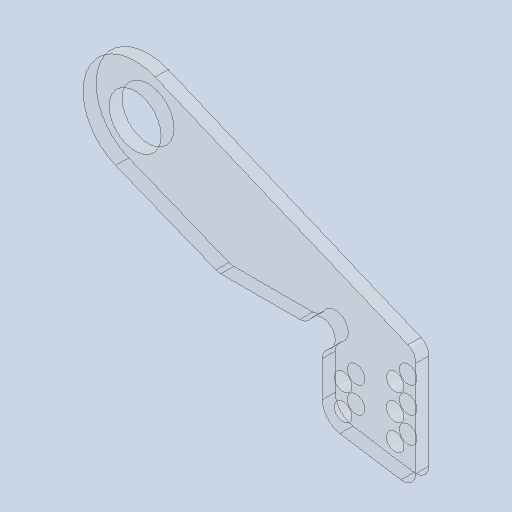
# Autodesk Inventor part: IntakePoly
Saved by Autodesk Inventor 2023 (Build 270158000, 158)
## iProperties
Created: 2022-11-06
Part Number: IntakePoly
Material: Polycarbonate, Smoke
Document SubType Name: Modeling
Designer: zac-h
Density: 1.2 g/cm^3
Appearance: Polycarbonate - Clear
Author: zac-h
Autodesk Inventor part; units mm, degrees
ref_plane "YZ Plane" through (0, 0, 0) normal (1, 0, 0) x (0, 1, 0)
ref_plane "XZ Plane" through (0, 0, 0) normal (0, 1, 0) x (-1, 0, 0)
ref_plane "XY Plane" through (0, 0, 0) normal (0, 0, 1) x (1, 0, 0)
sketch "Sketch1" plane through (0, 0, 0) normal (0, 0, 1) x (1, 0, 0)
  circle A0 centre (19.1135, 26.5479) radius 2.159 projected
  circle A1 centre (6.4135, 13.8479) radius 2.159 projected
  circle A2 centre (6.4135, 20.1979) radius 2.159 projected
  circle A3 centre (19.1135, 13.8479) radius 2.159 projected
  circle A4 centre (19.1135, 20.1979) radius 2.159 projected
  circle A5 centre (-11.4935, -25.7761) radius 2.159 projected
  circle A6 centre (-5.3048, -30.2218) radius 2.159 projected
  circle A7 centre (-17.6822, -21.3304) radius 2.159 projected
  arc A8 (2.921, 26.1944) -> (1.3335, 23.4448) centre (4.5085, 23.4448) ccw projected
  line L0 (1.3335, 23.4448) -> (1.3335, 14.8701) projected
  arc A9 (0.7371, 13.0177) -> (1.3335, 14.8701) centre (-1.8415, 14.8701) ccw projected
  line L1 (0.7371, 13.0177) -> (-21.808, -18.3666) projected
  arc A10 (-21.808, -18.3666) -> (-0.6209, -32.3394) centre (-11.4935, -25.7761) ccw projected
  line L2 (-0.6209, -32.3394) -> (23.7367, 8.0111) projected
  arc A11 (23.7367, 8.0111) -> (24.1935, 9.6519) centre (21.0185, 9.6519) ccw projected
  line L3 (24.1935, 9.6519) -> (24.1935, 32.9769) projected
  arc A12 (24.1935, 32.9769) -> (19.431, 35.7265) centre (21.0185, 32.9769) ccw projected
  line L4 (19.431, 35.7265) -> (2.921, 26.1944) projected
  circle A13 centre (21.0185, 9.6519) radius 3.175
  line L5 (1.3335, 14.8701) -> (1.3335, 13.8479)
  circle A14 centre (6.4135, 13.8479) radius 5.08
  line L6 (20.5313, 6.5145) -> (5.6339, 8.8281)
  circle A15 centre (-44.3865, 49.9375) radius 6.35
  circle A16 centre (-44.3865, 49.9375) radius 25.4 construction
  circle A17 centre (-11.4935, -25.7761) radius 82.55 construction
  circle A18 centre (-11.4935, -25.7761) radius 57.15 construction
  circle A19 centre (1.3335, 28.0719) radius 3.175
  line L7 (-1.8415, 28.0719) -> (-24.0665, 28.0719)
  circle A20 centre (-44.3865, 49.9375) radius 12.7
  line L8 (-24.0665, 28.0719) -> (-49.1272, 38.1555)
  line L9 (-39.4975, 61.6587) -> (22.2408, 35.9072)
  point P0 (0, 0)
  point P1 (1.6958, 24.9176)
  dimension "d10" = 6.35
  dimension "d3" = 12.7
  dimension "d4" = 50.8
  dimension "d5" = 114.3
  dimension "d6" = 45.72
  dimension "d8" = 25.4
  dimension "d12" = 1.524
  dimension "d13" = 25.4
  constraints: 10 end point, 7 point on circle, 7 tangent, 6 centre point, 6 coincident, 1 horizontal, 1 horizontal alignment, 1 vertical, 1 vertical alignment, 6 other
  measures "d3" diameter of A15
  measures "d4" diameter of A16
  measures "d5" diameter of A18
  measures "d6" distance from line of L0 A16.centre
  measures "d8" distance of point (1.333, 28.072) L7.end
  measures "d12" distance from line of A0.centre L7
  measures "d13" diameter of A20
extrude "Extrusion1" add sketch "Sketch1" along normal blind 3.175 contours A2 A14 L5 L0 A8 A19 L4 A12 L3 A13 A3 L6 | A2 A14 | A13 A3 A11 | L7 L8 A20 L9 A12 L4 A19 | A20 picked at (8.0498, 17.4208)
fillet "Fillet1" radius 3.175 3 edges at (1.6958, 24.9176, 1.5875) (-1.8415, 28.0719, 1.5875) (-24.0665, 28.0719, 1.5875)
body "Solid1"
